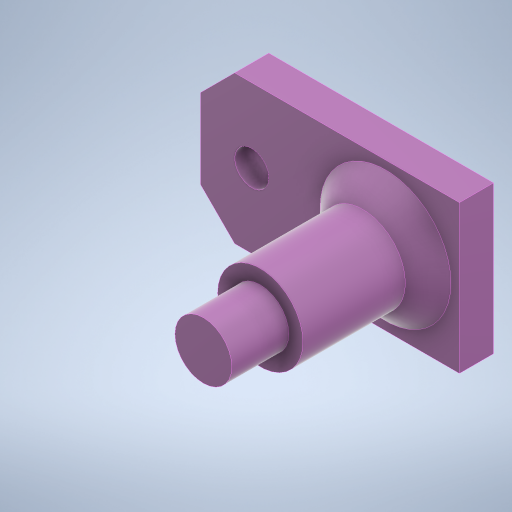
# Autodesk Inventor part: Концентратор
Saved by Autodesk Inventor 2024 (Build 280153020, 153B)
## iProperties
Created: 2023-06-09
Part Number: Концентратор
Material: Типовые
Document SubType Name: Modeling
Designer: Admin
Density: 1 g/cm^3
Appearance: По умолчанию
Author: Admin
Autodesk Inventor part; units mm, degrees
ref_plane "YZ Plane" through (0, 0, 0) normal (1, 0, 0) x (0, 1, 0)
ref_plane "XZ Plane" through (0, 0, 0) normal (0, 1, 0) x (-1, 0, 0)
ref_plane "XY Plane" through (0, 0, 0) normal (0, 0, 1) x (1, 0, 0)
sketch "Эскиз1" plane through (0, 0, 0) normal (0, 0, 1) x (1, 0, 0)
  line L0 (3, 0) -> (22.75, 0)
  line L1 (22.75, 0) -> (22.75, 13)
  line L2 (22.75, 13) -> (3, 13)
  line L3 (0, 10) -> (0, 3)
  circle A0 centre (16.25, 6.5) radius 8 construction
  circle A1 centre (16.25, 6.5) radius 2.5
  circle A2 centre (4.5, 6.5) radius 1.5
  line L4 (0, 6.5) -> (22.75, 6.5) construction
  circle A3 centre (4.5, 6.5) radius 2.75 construction
  line L5 (3, 13) -> (0, 10)
  line L6 (0, 3) -> (3, 0)
  circle A4 centre (16.25, 6.5) radius 3.75
  point P0 (0, 0)
  point P1 (0, 13)
  dimension "d0" = 16
  dimension "d3" = 3
  dimension "d6" = 5.5
  dimension "d7" = 1
  dimension "d9" = 3
  dimension "d10" = 3
  dimension "d11" = 3
  dimension "d12" = 3
  dimension "d13" = 7.5
  dimension "d23" = 6.5
  dimension "d24" = 6.5
  constraints: 14 end point, 6 point on line, 5 centre point, 3 coincident, 2 midpoint, 2 parallel, 1 horizontal, 1 perpendicular, 2 other
  measures "d0" diameter of A0
  measures "d3" distance edge to line of A2 L3
  measures "d6" diameter of A3
  measures "d9" distance of L2.end point (0, 13)
  measures "d10" distance of L3.start point (0, 13)
  measures "d11" distance of L3.end point (0, 0)
  measures "d12" distance of L0.start point (0, 0)
  measures "d13" diameter of A4
  measures "d23" distance from line of L2 A0.centre
  measures "d24" distance from line of L1 A0.centre
extrude "Выдавливание1" add sketch "Эскиз1" along normal blind 3 contours L6 L3 L5 L2 L1 L0
extrude "Выдавливание2" add sketch "Эскиз1" along normal blind 14 contours A4
extrude "Выдавливание3" add sketch "Эскиз1" along normal blind 19 contours A1
chamfer "Фаска1" distance 2 angle 45 1 edges at (12.5, 6.5, 3)
equation "\"d10\" = d9"
equation "\"d11\" = d9"
equation "\"d12\" = d11"
